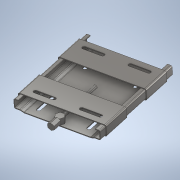
# Autodesk Inventor part: Base motor
Saved by Autodesk Inventor 2022.2 (Build 262287000, 287)
## iProperties
Part Number: Base motor
Material: Acciaio inossidabile
Document SubType Name: Lamiera
Designer: MDV
Mass: 4997.74 g
Surface Area: 3708.28 cm^2
Volume: 624.717 cm^3
Density: 8 g/cm^3
Appearance: Semilucidato
Sheet Metal Rule: Por defecto_mm
Author: MDV
Autodesk Inventor part; units mm, degrees
ref_plane "YZ Plane" through (0, 0, 0) normal (1, 0, 0) x (0, 1, 0)
ref_plane "XZ Plane" through (0, 0, 0) normal (0, 1, 0) x (-1, 0, 0)
ref_plane "XY Plane" through (0, 0, 0) normal (0, 0, 1) x (1, 0, 0)
sketch "Schizzo1" plane through (0, 0, 0) normal (0, 0, 1) x (1, 0, 0)
  line L0 (0, 0) -> (108.3772, 0)
  line L1 (142, 9) -> (142, 32)
  line L2 (137, 37) -> (127, 37)
  line L3 (137, 4) -> (123.6228, 4)
  line L4 (120.4605, 3.4868) -> (111.5395, 0.5132)
  arc A0 (108.3772, 0) -> (111.5395, 0.5132) centre (108.3772, 10) ccw
  arc A1 (123.6228, 4) -> (120.4605, 3.4868) centre (123.6228, -6) ccw
  arc A2 (142, 32) -> (137, 37) centre (137, 32) ccw
  arc A3 (137, 4) -> (142, 9) centre (137, 9) ccw
  line L5 (0, 3) -> (108.3772, 3)
  arc A4 (108.3772, 3) -> (110.5908, 3.3592) centre (108.3772, 10) ccw
  line L6 (110.5908, 3.3592) -> (119.5118, 6.3329)
  arc A5 (123.6228, 7) -> (119.5118, 6.3329) centre (123.6228, -6) ccw
  line L7 (123.6228, 7) -> (137, 7)
  arc A6 (137, 7) -> (139, 9) centre (137, 9) ccw
  line L8 (139, 9) -> (139, 32)
  arc A7 (139, 32) -> (137, 34) centre (137, 32) ccw
  line L9 (137, 34) -> (127, 34)
  line L10 (127, 34) -> (127, 37)
  line L11 (0, 0) -> (0, 43.1027)
  line L12 (0, 0) -> (-108.3772, 0)
  line L13 (-142, 9) -> (-142, 32)
  line L14 (-137, 37) -> (-127, 37)
  line L15 (-137, 4) -> (-123.6228, 4)
  line L16 (-120.4605, 3.4868) -> (-111.5395, 0.5132)
  arc A8 (-111.5395, 0.5132) -> (-108.3772, 0) centre (-108.3772, 10) ccw
  arc A9 (-120.4605, 3.4868) -> (-123.6228, 4) centre (-123.6228, -6) ccw
  arc A10 (-137, 37) -> (-142, 32) centre (-137, 32) ccw
  arc A11 (-142, 9) -> (-137, 4) centre (-137, 9) ccw
  line L17 (0, 3) -> (-108.3772, 3)
  arc A12 (-110.5908, 3.3592) -> (-108.3772, 3) centre (-108.3772, 10) ccw
  line L18 (-110.5908, 3.3592) -> (-119.5118, 6.3329)
  arc A13 (-119.5118, 6.3329) -> (-123.6228, 7) centre (-123.6228, -6) ccw
  line L19 (-123.6228, 7) -> (-137, 7)
  arc A14 (-139, 9) -> (-137, 7) centre (-137, 9) ccw
  line L20 (-139, 9) -> (-139, 32)
  arc A15 (-137, 34) -> (-139, 32) centre (-137, 32) ccw
  line L21 (-137, 34) -> (-127, 34)
  line L22 (-127, 34) -> (-127, 37)
  point P0 (142, 4)
  point P1 (142, 37)
  point P2 (122, 4)
  point P3 (110, 0)
  point P4 (-142, 4)
  point P5 (-142, 37)
  point P6 (-122, 4)
  point P7 (-110, 0)
  dimension "d2" = 15
  dimension "d3" = 33
  dimension "d4" = 12
  dimension "d6" = 20
  dimension "d7" = 142
  dimension "d8" = 10
  dimension "d9" = 5
  dimension "d63" = 37
  constraints: 46 end point, 32 point on circle, 26 symmetric about line, 16 centre point, 16 point on line, 8 tangent, 4 perpendicular, 2 equal radius, 2 horizontal, 2 parallel, 1 vertical, 16 other
  measures "d2" distance of point (142, 37) L2.end
  measures "d3" distance between parallel lines of L3 L2
  measures "d4" horizontal distance of point (110, 0) point (122, 4)
  measures "d6" distance of point (142, 4) point (122, 4)
  measures "d7" distance from line of L1 L0.start
  measures "d8" radius of A0
  measures "d9" radius of A2
  measures "d63" distance between parallel lines of L0 L2
extrude "Estrusione1" add sketch "Schizzo1" along normal blind 340
sketch "Schizzo2" plane through (-108.3772, 3, 0) normal (0, 1, 0) x (1, 0, 0)
  line L0 (32.1272, -92) -> (32.1272, -30)
  line L1 (19.6272, -30) -> (19.6272, -92)
  line L2 (19.6272, -92) -> (32.1272, -30) construction
  line L3 (32.1272, -92) -> (19.6272, -30) construction
  arc A0 (32.1272, -30) -> (19.6272, -30) centre (25.8772, -30) ccw
  arc A1 (19.6272, -92) -> (32.1272, -92) centre (25.8772, -92) ccw
  line L4 (108.3772, 68) -> (108.3772, -408) projected
  line L5 (184.6272, -92) -> (184.6272, -30)
  line L6 (197.1272, -30) -> (197.1272, -92)
  line L7 (197.1272, -92) -> (184.6272, -30) construction
  line L8 (184.6272, -92) -> (197.1272, -30) construction
  arc A2 (197.1272, -30) -> (184.6272, -30) centre (190.8772, -30) ccw
  arc A3 (184.6272, -92) -> (197.1272, -92) centre (190.8772, -92) ccw
  line L9 (216.7544, 0) -> (0, 0) projected
  line L10 (250.3772, 0) -> (250.3772, -340) projected
  line L11 (250.3772, -170) -> (-33.6228, -170)
  line L12 (-33.6228, 0) -> (-33.6228, -340) projected
  line L13 (32.1272, -248) -> (32.1272, -310)
  line L14 (19.6272, -310) -> (19.6272, -248)
  line L15 (19.6272, -248) -> (32.1272, -310) construction
  line L16 (32.1272, -248) -> (19.6272, -310) construction
  arc A4 (19.6272, -310) -> (32.1272, -310) centre (25.8772, -310) ccw
  arc A5 (32.1272, -248) -> (19.6272, -248) centre (25.8772, -248) ccw
  line L17 (184.6272, -248) -> (184.6272, -310)
  line L18 (197.1272, -310) -> (197.1272, -248)
  line L19 (197.1272, -248) -> (184.6272, -310) construction
  line L20 (184.6272, -248) -> (197.1272, -310) construction
  arc A6 (184.6272, -310) -> (197.1272, -310) centre (190.8772, -310) ccw
  arc A7 (197.1272, -248) -> (184.6272, -248) centre (190.8772, -248) ccw
  point P0 (25.8772, -61)
  point P1 (190.8772, -61)
  point P2 (25.8772, -279)
  point P3 (190.8772, -279)
  dimension "Quota_P" = 165
  constraints: 34 end point, 21 symmetric about line, 16 point on circle, 10 midpoint, 8 centre point, 4 tangent, 2 parallel, 1 vertical alignment, 7 other
  measures "Quota_P" distance of A2.centre A0.centre
extrude "Estrusione2" cut sketch "Schizzo2" against normal blind 210
sketch "Schizzo3" plane through (-137, 37, 0) normal (0, 1, 0) x (1, 0, 0)
  line L0 (-5, 0) -> (-5, -340) projected
  line L1 (279, 0) -> (279, -340) projected
  line L2 (-5, -309) -> (279, -309)
  line L3 (279, -309) -> (279, -214)
  line L4 (279, -214) -> (-5, -214)
  line L5 (-5, -214) -> (-5, -309)
  line L6 (-5, 0) -> (-5, -340) projected
  line L7 (279, -25) -> (-5, -25)
  line L8 (-5, -25) -> (-5, -120)
  line L9 (-5, -120) -> (279, -120)
  line L10 (279, -120) -> (279, -25)
  line L11 (244, -275.75) -> (182, -275.75)
  line L12 (182, -288.25) -> (244, -288.25)
  line L13 (244, -275.75) -> (182, -288.25) construction
  line L14 (182, -275.75) -> (244, -288.25) construction
  arc A0 (244, -288.25) -> (244, -275.75) centre (244, -282) ccw
  arc A1 (182, -275.75) -> (182, -288.25) centre (182, -282) ccw
  line L15 (137, -120) -> (137, -214)
  line L16 (137, -167) -> (203.7914, -167)
  line L17 (30, -275.75) -> (92, -275.75)
  line L18 (92, -288.25) -> (30, -288.25)
  line L19 (30, -275.75) -> (92, -288.25) construction
  line L20 (92, -275.75) -> (30, -288.25) construction
  arc A2 (30, -275.75) -> (30, -288.25) centre (30, -282) ccw
  arc A3 (92, -288.25) -> (92, -275.75) centre (92, -282) ccw
  line L21 (244, -58.25) -> (182, -58.25)
  line L22 (182, -45.75) -> (244, -45.75)
  line L23 (244, -58.25) -> (182, -45.75) construction
  line L24 (182, -58.25) -> (244, -45.75) construction
  arc A4 (244, -58.25) -> (244, -45.75) centre (244, -52) ccw
  arc A5 (182, -45.75) -> (182, -58.25) centre (182, -52) ccw
  line L25 (92, -45.75) -> (30, -45.75)
  line L26 (30, -58.25) -> (92, -58.25)
  line L27 (92, -58.25) -> (30, -45.75) construction
  line L28 (30, -58.25) -> (92, -45.75) construction
  arc A6 (92, -58.25) -> (92, -45.75) centre (92, -52) ccw
  arc A7 (30, -45.75) -> (30, -58.25) centre (30, -52) ccw
  point P0 (137, 0)
  point P1 (213, -282)
  point P2 (61, -282)
  point P3 (213, -52)
  point P4 (61, -52)
  dimension "Quota_L" = 95
  dimension "d54" = 95
  dimension "d55" = 12.5
  dimension "Quota_N" = 62
  dimension "Quota_C" = 27
  dimension "Quota_M" = 90
  dimension "InterasseForiMotore" = 230
  dimension "InizioViteTenditore" = 25
  constraints: 52 end point, 21 symmetric about line, 16 point on circle, 11 midpoint, 8 centre point, 5 parallel, 4 horizontal, 4 point on line, 4 tangent, 2 perpendicular, 6 other
  measures "Quota_L" distance between parallel lines of L2 L4
  measures "d54" distance between parallel lines of L9 L7
  measures "d55" distance between parallel lines of L11 L12
  measures "Quota_N" distance of A1.centre A0.centre
  measures "Quota_C" distance from line of L2 A0.centre
  measures "Quota_M" distance of A3.centre A1.centre
  measures "InterasseForiMotore" distance of A0.centre A4.centre
  measures "InizioViteTenditore" distance from line of point (137, 0) L7
extrude "Estrusione3" add sketch "Schizzo3" along normal blind 3 contours L7 L1 L9 L0 | L4 L1 L2 L0
sketch "Schizzo4" plane through (142, 37, 309) normal (1, 0, 0) x (0, 1, 0)
  line L0 (0, -95) -> (0, 0)
  line L1 (0, 0) -> (-33, 0)
  line L2 (-33, 0) -> (-33, -95)
  line L3 (-33, -95) -> (0, -95)
  constraints: 4 end point, 4 other
edge flange "Flangia1" height 36 angle 90 thickness 3 bend radius 3 thickness toward (1, 0, 0) relief tear relief width 3 relief depth 1.5 corner gap 3 corner form 0 edges at (142, 37, 261.5) (142, 37, 72.5) (-142, 37, 72.5) wall of the first edge with corners at (142, 37, 214) (142, 37, 309) (142, 4, 309) (142, 4, 214)
bend "Piega (Bend)1"
corner "Angolo1"
sketch "Schizzo5" plane through (-142, 37, 214) normal (-1, 0, 0) x (0, -1, 0)
  line L0 (0, 95) -> (0, 0)
  line L1 (0, 0) -> (33, 0)
  line L2 (33, 0) -> (33, 95)
  line L3 (33, 95) -> (0, 95)
  constraints: 4 end point, 4 other
edge flange "Flangia2" height 36 angle 90 thickness 3 bend radius 3 thickness toward (-1, 0, 0) relief tear relief width 3 relief depth 1.5 edges at (-142, 37, 261.5) wall of the first edge with corners at (-142, 37, 309) (-142, 37, 214) (-142, 4, 214) (-142, 4, 309)
bend "Piega (Bend)2"
corner "Angolo2"
sketch "Schizzo6" plane through (-142, 4, 214) normal (0, -1, 0) x (1, 0, 0)
  line L0 (0, 95) -> (0, 0)
  line L1 (0, 0) -> (17, 0)
  line L2 (17, 0) -> (17, 95)
  line L3 (17, 95) -> (0, 95)
  constraints: 4 end point, 4 other
edge flange "Flangia3" height 20 angle 90 thickness 3 bend radius 3 thickness toward (0, -1, 0) relief tear relief width 3 relief depth 1.5 corner gap 3 corner form 0 edges at (-142, 4, 261.5) (142, 4, 261.5) (142, 4, 72.5) (-142, 4, 72.5) wall of the first edge with corners at (-142, 4, 309) (-142, 4, 214) (-125, 4, 214) (-125, 4, 309)
bend "Piega (Bend)3"
corner "Angolo3"
fillet "Arrotondamento angolo1" radius 5 8 edges at (-125, 2.5, 214) (-125, 2.5, 309) (125, 2.5, 120) (125, 2.5, 25) (-125, 2.5, 120) (-125, 2.5, 25) (125, 2.5, 214) (125, 2.5, 309)
sketch "Schizzo7" plane through (-137, 37, 0) normal (0, -1, 0) x (1, 0, 0)
  line L0 (124.2983, 105) -> (130.6491, 116)
  line L1 (130.6491, 116) -> (143.3509, 116)
  line L2 (143.3509, 116) -> (149.7017, 105)
  line L3 (149.7017, 105) -> (143.3509, 94)
  line L4 (143.3509, 94) -> (130.6491, 94)
  line L5 (130.6491, 94) -> (124.2983, 105)
  line L6 (10, 120) -> (264, 120) projected
  line L7 (28.6228, 0) -> (245.3772, 0) projected
  point P0 (137, 0)
  point P1 (137, 105)
  point P2 (137, 0)
  dimension "d64" = 22
  dimension "d65" = 15
  constraints: 12 end point, 1 midpoint, 1 parallel, 1 vertical alignment, 13 other
  measures "d64" distance between parallel lines of L0 L3
  measures "d65" distance from line of L6 point (137, 105)
extrude "Estrusione4" add sketch "Schizzo7" along normal up to next
sketch "Schizzo8" plane through (-108.3772, 3, 0) normal (0, 1, 0) x (1, 0, 0)
  line L0 (93.3661, -13) -> (100.8717, 0)
  line L1 (100.8717, 0) -> (115.8828, 0)
  line L2 (115.8828, 0) -> (123.3883, -13)
  line L3 (123.3883, -13) -> (115.8828, -26)
  line L4 (115.8828, -26) -> (100.8717, -26)
  line L5 (100.8717, -26) -> (93.3661, -13)
  line L6 (216.7544, 0) -> (0, 0) projected
  point P0 (108.3772, 0)
  point P1 (108.3772, -13)
  point P2 (108.3772, 0)
  dimension "d68" = 26
  constraints: 12 end point, 1 collinear, 1 midpoint, 1 vertical alignment, 13 other
  measures "d68" distance between parallel lines of L4 L1
extrude "Estrusione5" add sketch "Schizzo8" along normal blind 22
sketch "Schizzo9" plane through (0, 0, 0) normal (0, 0, -1) x (-1, 0, 0)
  line L0 (0, 27.7017) -> (11, 21.3509)
  line L1 (11, 21.3509) -> (11, 8.6491)
  line L2 (11, 8.6491) -> (0, 2.2983)
  line L3 (0, 2.2983) -> (-11, 8.6491)
  line L4 (-11, 8.6491) -> (-11, 21.3509)
  line L5 (-11, 21.3509) -> (0, 27.7017)
  line L6 (7.5056, 3) -> (108.3772, 3) projected
  point P0 (0, 0)
  point P1 (0, 15)
  dimension "Quota_Ch" = 22
  dimension "d72" = 12
  constraints: 12 end point, 13 other
  measures "Quota_Ch" distance between parallel lines of L4 L1
  measures "d72" distance from line of L6 point (0, 15)
extrude "Estrusione6" add sketch "Schizzo9" along normal blind 30
sketch "Schizzo10" plane through (0, 0, 0) normal (0, 0, -1) x (-1, 0, 0)
  circle A0 centre (0, 15) radius 6
  line L0 (7.5056, 3) -> (108.3772, 3) projected
  point P0 (0, 0)
  dimension "d75" = 12
  dimension "d76" = 12
  constraints: 1 centre point
  measures "d75" diameter of A0
  measures "d76" distance from line of L0 A0.centre
extrude "Estrusione7" add sketch "Schizzo10" against normal blind 180
thread "Filettatura1" size "M12x1.75" class "6g" standard "ANSI Metric M Profile" full length
thread "Filettatura2" size "M12x1.75" class "6g" standard "ANSI Metric M Profile" full length
sketch "Schizzo11" plane through (-127, 37, 309) normal (0, 0, 1) x (1, 0, 0)
  line L0 (272, -30) -> (272, -3) projected
  line L1 (-18, -3) -> (-18, -30) projected
  line L2 (18.6228, -37) -> (235.3772, -37) projected
  line L3 (-12, 3) -> (266, 3) projected
  line L4 (234, 0) -> (234, 3) projected
  point P0 (127, -37)
  point P1 (335, -22)
  point P2 (272, -3)
  point P3 (272, -33)
  point P4 (-18, -33)
  point P5 (272, -3)
  point P6 (162, 0)
  dimension "Quota_O" = 38
  constraints: 2 other
equation "\"d54\" = Quota_L"
equation "\"d76\" = d72"
equation "\"d23\" = LarghezzaScaricoPiega"
equation "\"d24\" = ProfonditàScaricoPiega"
equation "\"d25\" = ResiduoMinimo"
equation "\"d26\" = RaggioPiega"
equation "\"d29\" = RaggioPiega"
equation "\"d30\" = DimensioniScaricoAngolo"
equation "\"d31\" = DimensioneGioco"
equation "\"d32\" = Dimensione_raggio_Jacobi"
equation "\"d33\" = LarghezzaScaricoPiega"
equation "\"d34\" = ProfonditàScaricoPiega"
equation "\"d35\" = ResiduoMinimo"
equation "\"d36\" = RaggioPiega"
equation "\"d39\" = RaggioPiega"
equation "\"d40\" = DimensioniScaricoAngolo"
equation "\"d41\" = DimensioneGioco"
equation "\"d42\" = Dimensione_raggio_Jacobi"
equation "\"d43\" = LarghezzaScaricoPiega"
equation "\"d44\" = ProfonditàScaricoPiega"
equation "\"d45\" = ResiduoMinimo"
equation "\"d46\" = RaggioPiega"
equation "\"d49\" = RaggioPiega"
equation "\"d50\" = DimensioniScaricoAngolo"
equation "\"d51\" = DimensioneGioco"
equation "\"d52\" = Dimensione_raggio_Jacobi"
equation "\"RaggioPiega\" = Spessore"
equation "\"LarghezzaScaricoPiega\" = Spessore"
equation "\"ProfonditàScaricoPiega\" = 0.5 * Spessore"
equation "\"DimensioniScaricoAngolo\" = 4 * Spessore"
equation "\"ResiduoMinimo\" = 2 * Spessore"
equation "\"RaggioTransizione\" = RaggioPiega"
equation "\"Dimensione_raggio_Jacobi\" = RaggioPiega"
equation "\"DimensioneGioco\" = Spessore"
equation "\"Spessore\" = 3"
